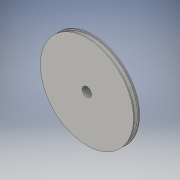
# Autodesk Inventor part: wheel
Saved by Autodesk Inventor 2016 (Build 200138000, 138)
## iProperties
Created: 2019-02-13
Part Number: wheel
Material: Generic
Document SubType Name: Modeling
Designer: reesem783
Density: 1 g/cm^3
Appearance: Default
Author: reesem783
Autodesk Inventor part; units mm, degrees
ref_plane "YZ Plane" through (0, 0, 0) normal (1, 0, 0) x (0, 1, 0)
ref_plane "XZ Plane" through (0, 0, 0) normal (0, 1, 0) x (-1, 0, 0)
ref_plane "XY Plane" through (0, 0, 0) normal (0, 0, 1) x (1, 0, 0)
sketch "Sketch1" plane through (0, 0, 0) normal (1, 0, 0) x (0, 1, 0)
  line L0 (0, 0) -> (0, -2.54)
  line L1 (0, -2.54) -> (-19.1008, -2.54)
  line L2 (-19.1008, -2.54) -> (-19.1008, -2.159)
  line L3 (0, 0) -> (-19.1008, 0)
  line L4 (-19.1008, 0) -> (-19.1008, -0.381)
  line L5 (-19.1008, -2.159) -> (-18.5928, -2.159)
  line L6 (-19.1008, -0.381) -> (-18.5928, -0.381)
  arc A0 (-18.5928, -2.159) -> (-18.5928, -0.381) centre (-18.5928, -1.27) ccw
  dimension "w" = 2.54
  dimension "d1" = 19.1008
  dimension "a" = 0.381
  dimension "d17" = 0.381
  dimension "d18" = 0.889
  constraints: 14 end point, 3 horizontal, 3 perpendicular, 2 point on circle, 1 centre point, 1 tangent, 1 vertical
  measures "w" distance of L0.start L0.end
  measures "d1" distance of L0.end L1.end
  measures "a" distance of L1.end L2.end
  measures "d17" distance of L3.end L4.end
  measures "d18" radius of A0
revolve "Revolution1" add sketch "Sketch1" angle 360 about axis through (0, 0, 0) along (0, 0, -1)
sketch "Sketch2" plane through (0, 0, 0) normal (0, 0, 1) x (1, 0, 0)
  point P0 (0, 0)
  point P1 (0, 0)
  constraints: 1 coincident
hole "Hole1" at (0, 0, 0) direction (0, 0, -1) diameter 3.81 end through all clearance for "Flat Head Machine Screw (82)" size "#6" standard "Ansi Unified Screw Threads"
equation "\"d17\" = a"
body "Solid1"
